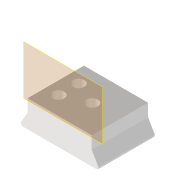
# Autodesk Inventor part: 10_Cassete_Slide
Saved by Autodesk Inventor 2022 (Build 260153000, 153)
## iProperties
Created: 2023-02-13
Part Number: 10_Cassete_Slide
Material: Generisch
Document SubType Name: Modeling
Designer: diederichbenedict
Density: 1 g/cm^3
Appearance: Vorgabe
Author: diederichbenedict
Autodesk Inventor part; units mm, degrees
ref_plane "YZ Plane" through (0, 0, 0) normal (1, 0, 0) x (0, 1, 0)
ref_plane "XZ Plane" through (0, 0, 0) normal (0, 1, 0) x (-1, 0, 0)
ref_plane "Arbeitsebene1" through (0, 0, 0) normal (0, 0, 1) x (1, 0, 0)
sketch "Skizze1" plane through (0, 0, 0) normal (0, 0, 1) x (1, 0, 0)
  arc A0 (-53, 5.4) -> (-47.2, -0.4) centre (-47.2, 5.4) ccw projected
  line L0 (-53, -5.4) -> (-53, 5.4) projected
  line L1 (-35.6871, -5.4) -> (-53, -5.4) projected
  line L2 (-35.6871, -0.4) -> (-35.6871, -5.4) projected
  line L3 (-47.2, -0.4) -> (-35.6871, -0.4) projected
  line L4 (-67.0006, -5.9) -> (-67.0006, -9.9) projected
  line L5 (-31.7506, -5.4) -> (-31.7506, -10.4) projected
  line L6 (-33.0006, -5.9) -> (-33.0006, -9.9) construction
  line L7 (-32.5561, -5.4) -> (-32.5561, -10.4) projected
  line L8 (-51.4006, -5.4) -> (-51.4006, 4.6)
  line L9 (-48.6006, -5.4) -> (-48.6006, 2.412)
  line L10 (-35.6871, -5.4) -> (-53.0408, -5.4)
  line L11 (-53.0408, -5.4) -> (-53.0408, -8.4)
  line L12 (-53.0408, -8.4) -> (-37.6871, -8.4)
  line L13 (-37.6871, -8.4) -> (-37.6871, -5.4)
  line L14 (-53.0408, -8.4) -> (-55.0408, -11.8641)
  line L15 (-53.0408, -8.4) -> (-49.0408, -8.4) construction
  line L16 (-55.0408, -11.8641) -> (-35.6871, -11.8641)
  line L17 (-35.6871, -11.8641) -> (-37.6871, -8.4)
  point P0 (0, 0)
  dimension "d0" = 3
  dimension "d1" = 4
  dimension "d2" = 120
  dimension "d3" = 60
  dimension "d14" = 2
  constraints: 20 end point, 3 horizontal, 2 parallel, 2 vertical, 1 equal length, 1 perpendicular, 1 point on line, 4 other
  measures "d0" distance of L11.end L10.end
  measures "d1" distance of L11.end L14.end
  measures "d2" angle of L14 L15
  measures "d3" angle of L17 L16
  measures "d14" distance between parallel lines of L2 L13
ref_plane "Arbeitsebene2" through (-53, -5.4, -13.5) normal (0, 0, -1) x (0, 1, 0)
extrude "Extrusion1" add sketch "Skizze1" against normal up to surface (13.5 mm away) contours L1 L13 L12 L11 L10 | L12 L17 L16 L14
fillet "Rundung1" radius 0.5 4 edges at (-55.0408, -11.8641, -6.75) (-35.6871, -11.8641, -6.75) (-53.0408, -8.4, -6.75) (-37.6871, -8.4, -6.75)
sketch "Skizze2" plane through (-54.1748, -11.8641, 0) normal (0, -1, 0) x (1, 0, 0)
  circle A0 centre (9.8312, -6.75) radius 1.4 projected
  circle A1 centre (4.1742, -4.35) radius 1.4 projected
  line L0 (-0.6431, -6.75) -> (20.1351, -6.75)
  circle A2 centre (4.1742, -9.15) radius 1.4
  point P0 (54.1748, 0)
  constraints: 2 end point, 1 centre point, 1 horizontal, 1 symmetric about line, 1 other
hole "Bohrung1" at (-50.0006, -11.8641, -4.35) at (-44.3436, -11.8641, -6.75) at (-50.0006, -11.8641, -9.15) direction (0, 1, 0) diameter 2.8 depth 14 tip angle 118 counterbore diameter 6.5 counterbore depth 3
